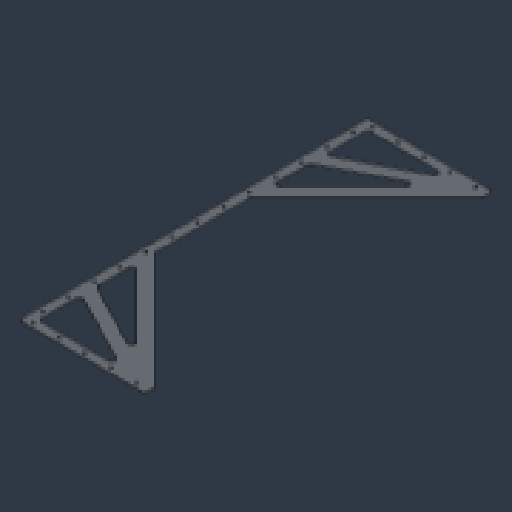
# Autodesk Inventor part: TOP_INTAKE_LEXAN
Saved by Autodesk Inventor 2026 (Build 300175050, 175E)
## iProperties
Created: 2026-04-02
Part Number: TOP_INTAKE_LEXAN
Material: Polycarbonate, PC 1000, Clear
Document SubType Name: Sheet Metal
Designer: 4aida
Density: 1.20131 g/cm^3
Sheet Metal Rule: Default_mm
Appearance: Lexan (Clear)
Mass: 180.794 g
Surface Area: 1075.56 cm^2
Volume: 150.498 cm^3
Author: 4aida
Autodesk Inventor part; units mm, degrees
ref_plane "YZ Plane" through (0, 0, 0) normal (1, 0, 0) x (0, 1, 0)
ref_plane "XZ Plane" through (0, 0, 0) normal (0, 1, 0) x (-1, 0, 0)
ref_plane "XY Plane" through (0, 0, 0) normal (0, 0, 1) x (1, 0, 0)
sketch "Sketch1" plane through (0, 0, 0) normal (0, 1, 0) x (-1, 0, 0)
  line L0 (-123.825, -342.392) -> (123.825, -342.392)
  line L1 (123.825, -342.392) -> (123.825, 342.392)
  line L2 (123.825, 342.392) -> (-123.825, 342.392)
  line L3 (-123.825, 342.392) -> (-123.825, -342.392)
  line L4 (-123.825, -342.392) -> (123.825, 342.392) construction
  line L5 (123.825, -342.392) -> (-123.825, 342.392) construction
  line L6 (104.775, -323.342) -> (104.775, 323.342)
  line L7 (104.775, 323.342) -> (-123.825, 323.342)
  line L8 (104.775, -323.342) -> (-123.825, -323.342)
  line L9 (-123.825, -323.342) -> (104.775, -94.742)
  line L10 (104.775, -130.663) -> (-87.904, -323.342)
  line L11 (-58.7715, -294.2096) -> (104.775, -209.0726)
  line L12 (104.775, -237.7081) -> (-59.7261, -323.342)
  line L13 (104.775, -223.3904) -> (-123.825, -342.392) construction
  line L14 (104.775, 0) -> (103.1663, 0)
  line L15 (-123.825, 323.342) -> (104.775, 94.742)
  line L16 (104.775, 130.663) -> (-87.904, 323.342)
  line L17 (-58.7715, 294.2096) -> (104.775, 209.0726)
  line L18 (104.775, 237.7081) -> (-59.7261, 323.342)
  point P0 (0, 0)
  point P1 (104.775, 223.3904)
  point P2 (104.775, 94.742)
  point P3 (104.775, 130.663)
  point P4 (104.775, 209.0726)
  point P5 (-59.7261, 323.342)
  dimension "d0" = 19.05
  dimension "d1" = 19.05
  dimension "d2" = 19.05
  dimension "d4" = 228.6
  dimension "d5" = 646.684
  dimension "d6" = 25.4
  dimension "d7" = 45
  dimension "d9" = 25.4
  dimension "d10" = 12.7
  dimension "d11" = 17.5
  measures "d0" distance between parallel lines of L1 L6
  measures "d1" distance between parallel lines of L7 L2
  measures "d2" distance between parallel lines of L0 L8
  measures "d4" distance between parallel lines of L3 L6
  measures "d5" distance of L6.start L6.end
  measures "d6" distance between parallel lines of L10 L9
  measures "d7" angle of L8 L10
  measures "d9" distance between parallel lines of L12 L11
  measures "d10" distance between parallel lines of L13 L11
  measures "d11" angle of L11 L10
extrude "Plate1" add sketch "Sketch1" along normal blind 3.175 contours L3 L8 L6 L7 L2 L1 L0 | L9 L6 L10 L8 | L7 L16 L6 L15 | L10 L11 L6 L12 L8 | L7 L18 L6 L17 L16
fillet "Corner Round1" radius 6.35 20 edges at (-123.825, 1.5875, 342.392) (123.825, 1.5875, 342.392) (123.825, 1.5875, 323.342) (59.7261, 1.5875, 323.342) (58.7715, 1.5875, 294.2096) (-104.775, 1.5875, 237.7081) (-104.775, 1.5875, 323.342) (-104.775, 1.5875, 209.0726) (-104.775, 1.5875, 130.663) (-104.775, 1.5875, 94.742) (-104.775, 1.5875, -94.742) (-104.775, 1.5875, -130.663) (-104.775, 1.5875, -209.0726) (-104.775, 1.5875, -237.7081) (58.7715, 1.5875, -294.2096) (123.825, 1.5875, -323.342) (123.825, 1.5875, -342.392) (-123.825, 1.5875, -342.392) (59.7261, 1.5875, -323.342) (-104.775, 1.5875, -323.342)
sketch "Sketch2" plane through (0, 0, 0) normal (0, -1, 0) x (1, 0, 0)
  line L0 (-117.475, 342.392) -> (117.475, 342.392) projected
  line L1 (123.825, 336.042) -> (123.825, 325.9723) projected
  line L2 (-104.775, 92.1117) -> (-104.775, -92.1117) projected
  point P0 (0, 0)
  point P1 (98.425, 332.867)
  point P2 (47.625, 332.867)
  point P3 (-3.175, 332.867)
  point P4 (-53.975, 332.867)
  point P5 (-104.775, 332.867)
  point P6 (-155.575, 332.867)
  point P7 (-114.3, 0)
  point P8 (-104.775, 0)
  point P9 (-114.3, 50.8)
  point P10 (-114.3, 101.6)
  point P11 (-114.3, 152.4)
  point P12 (-114.3, 203.2)
  point P13 (-114.3, 254)
  point P14 (-114.3, 304.8)
  dimension "d14" = 9.525
  dimension "d15" = 25.4
  dimension "d18" = 50.8
  dimension "d23" = 9.525
  dimension "d26" = 50.8
  constraints: 1 horizontal, 1 horizontal alignment, 1 midpoint, 1 vertical, 11 other
  measures "d14" distance from line of L0 point (98.425, 332.867)
  measures "d15" distance from line of L1 point (98.425, 332.867)
  measures "d18" distance of point (98.425, 332.867) point (47.625, 332.867)
  measures "d23" distance from line of L2 point (-114.3, 0)
  measures "d26" distance of point (-114.3, 0) point (-114.3, 50.8)
hole "Hole1" at (98.425, 0, 332.867) at (47.625, 0, 332.867) at (-3.175, 0, 332.867) at (-53.975, 0, 332.867) at (-104.775, 0, 332.867) at (-155.575, 0, 332.867) at (-114.3, 0, 0) at (-114.3, 0, 50.8) at (-114.3, 0, 101.6) at (-114.3, 0, 152.4) at (-114.3, 0, 203.2) at (-114.3, 0, 254) at (-114.3, 0, 304.8) direction (0, 1, 0) diameter 5.105 end through all clearance for "Flat Head Machine Screw (82)" size "#10" standard "Ansi Unified Screw Threads"
mirror "Mirror1" about plane through (0, 0, 0) normal (0, 0, 1) of "Hole1"
equation "\"d1\" = d0"
equation "\"d2\" = d0"
equation "\"d9\" = d6"
equation "\"d10\" = 0.5 * d9"
equation "\"d36\" = Thickness"
equation "\"d12\" = Thickness"
equation "\"BendRadius\" = Thickness"
equation "\"BendReliefWidth\" = Thickness"
equation "\"BendReliefDepth\" = 0.5 * Thickness"
equation "\"CornerReliefSize\" = 4 * Thickness"
equation "\"MinimumRemnant\" = 2 * Thickness"
equation "\"TransitionRadius\" = BendRadius"
equation "\"JacobiRadiusSize\" = BendRadius"
equation "\"GapSize\" = Thickness"
equation "\"Thickness\" = 3.175"
body "Solid1"
